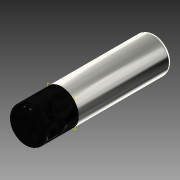
# Autodesk Inventor part: 739136_AA
Saved by Autodesk Inventor 2018 (Build 220112000, 112)
## iProperties
Category: Electrical Accessories
Company: Autodesk Inc.
Created: 2014-11-27
Part Number: 739136_AA
Material: Generic
Document SubType Name: Modeling
Designer: Tetrix
Density: 1 g/cm^3
Appearance: Default
Catalog Web Link: http://www.tetrixrobotics.com/AA_Battery_Holder
Vendor: Tetrix
Author: Autodesk Inc.
Autodesk Inventor part; units mm, degrees
ref_plane "YZ Plane" through (0, 0, 0) normal (1, 0, 0) x (0, 1, 0)
ref_plane "XZ Plane" through (0, 0, 0) normal (0, 1, 0) x (-1, 0, 0)
ref_plane "XY Plane" through (0, 0, 0) normal (0, 0, 1) x (1, 0, 0)
sketch "Sketch1" plane through (0, 0, 0) normal (0, 1, 0) x (-1, 0, 0)
  circle A0 centre (0, 0) radius 7
  dimension "d0" = 14
  constraints: 1 centre point, 1 coincident
  measures "d0" diameter of A0
extrude "Extrusion1" add sketch "Sketch1" along normal blind 53
fillet "Fillet1" radius 2 2 edges at (7, 0, 0) (7, 53, 0)
ref_plane "Work Plane1" through (0, 15, 0) normal (0, -1, 0) x (1, 0, 0)
split_face "Split1"
body "Solid1"
